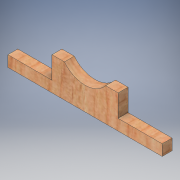
# Autodesk Inventor part: Soporte para Motor
Saved by Autodesk Inventor 2016 SP2 (Build 200236200, 236)
## iProperties
Created: 2017-06-26
Part Number: Soporte para Motor
Material: Abedul
Document SubType Name: Modeling
Designer: ssant
Density: 0.512 g/cm^3
Appearance: Abedul - Natural brillo medio
Author: ssant
Autodesk Inventor part; units mm, degrees
ref_plane "YZ Plane" through (0, 0, 0) normal (1, 0, 0) x (0, 1, 0)
ref_plane "XZ Plane" through (0, 0, 0) normal (0, 1, 0) x (-1, 0, 0)
ref_plane "XY Plane" through (0, 0, 0) normal (0, 0, 1) x (1, 0, 0)
sketch "Boceto1" plane through (0, 0, 0) normal (0, 0, 1) x (1, 0, 0)
  line L0 (30, 15) -> (30, -5)
  line L1 (30, -15) -> (-30, -15)
  line L2 (-30, -5) -> (-30, 15)
  arc A0 (-18.735, 15) -> (18.735, 15) centre (0, 30) ccw
  line L3 (-30, 15) -> (-18.735, 15)
  line L4 (18.735, 15) -> (30, 15)
  line L5 (-30, -15) -> (-70, -15)
  line L6 (-70, -15) -> (-70, -5)
  line L7 (-70, -5) -> (-30, -5)
  line L8 (30, -15) -> (70, -15)
  line L9 (30, -15) -> (70, -15) construction
  line L10 (70, -15) -> (70, -5)
  line L11 (70, -5) -> (30, -5)
  point P0 (0, 0)
  point P1 (-30, 0)
  point P2 (0, -15)
  point P3 (0, 6)
  dimension "d0" = 60
  dimension "d1" = 30
  dimension "d3" = 45
  dimension "d4" = 24
  dimension "d5" = 40
  dimension "d6" = 10
  dimension "d7" = 40
  constraints: 24 end point, 6 perpendicular, 5 horizontal, 3 parallel, 3 point on circle, 3 vertical alignment, 1 centre point, 1 collinear, 1 horizontal alignment, 1 midpoint, 1 point on line
  measures "d0" distance of L1.start L1.end
  measures "d1" distance of L0.start L1.start
  measures "d3" distance of point (0, -15) A0.centre
  measures "d4" radius of A0
  measures "d5" distance of L1.end L5.end
  measures "d6" distance of L5.end L6.end
  measures "d7" distance of L1.start L8.end
extrude "Extrusión1" add sketch "Boceto1" against normal blind 9
sketch "Boceto2" plane through (-70, -15, 0) normal (0, -1, 0) x (1, 0, 0)
  line L0 (0, 0) -> (140, 0) projected
  line L1 (0, 0) -> (0, -9) projected
  line L2 (140, -9) -> (0, -9) projected
  line L3 (140, 0) -> (140, -9) projected
  line L4 (100, 0) -> (100, -9) projected
  line L5 (40, 0) -> (40, -9) projected
  point P0 (70, 0)
  point P1 (47.5, -4.5)
  point P2 (92.5, -4.5)
  dimension "d11" = 4.5
  dimension "d12" = 4.5
  dimension "d13" = 7.5
  dimension "d14" = 7.5
  measures "d11" distance from line of L2 point (92.5, -4.5)
  measures "d12" distance from line of L2 point (47.5, -4.5)
  measures "d13" distance from line of L5 point (47.5, -4.5)
  measures "d14" distance from line of L4 point (92.5, -4.5)
hole "Agujero1" at (-22.5, -15, -4.5) at (22.5, -15, -4.5) direction (0, 1, 0) diameter 5 depth 20
